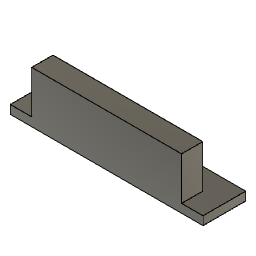
Insert (Autodesk Fusion 360 design; units mm, degrees)
Autodesk Fusion 360 part; units mm, degrees
sketch "Sketch1" plane through (0, 0, 0) normal (0, 0, 1) x (1, 0, 0)
  line L0 (0, 0) -> (44.95, 0)
  line L1 (44.95, 0) -> (44.95, 14.95)
  line L2 (44.95, 14.95) -> (0, 14.95)
  line L3 (0, 14.95) -> (0, 0)
  line L4 (5, 5) -> (39.95, 5)
  line L5 (39.95, 5) -> (39.95, 9.95)
  line L6 (39.95, 9.95) -> (5, 9.95)
  line L7 (5, 9.95) -> (5, 5)
  dimension "d1" = 44.95
  dimension "d2" = 14.95
  dimension "d3" = 34.95
  dimension "d4" = 4.95
  dimension "d5" = 5
  dimension "d6" = 5
  constraint horizontal L0
  constraint vertical L1
  constraint horizontal L2
  constraint vertical L3
  constraint coincident L0.start L3.end
  constraint horizontal L4
  constraint vertical L5
  constraint horizontal L6
  constraint vertical L7
  measures "d1" distance of L0.start L0.end
  measures "d2" distance of L0.start L2.end
  measures "d3" distance of L4.start L4.end
  measures "d4" distance of L4.start L6.end
  measures "d5" distance of L2 L6
  measures "d6" distance of L3 L7
extrude "Extrude1" add sketch "Sketch1" along normal blind 12 contours L4 L5 L6 L7
extrude "Extrude2" add sketch "Sketch1" along normal blind 2
sketch "Sketch2" plane through (0, 0, 2) normal (0, 0, 1) x (-1, 0, 0)
  line L0 (-5, -5) -> (-5, -9.95)
  line L1 (-5, -9.95) -> (-39.95, -9.95)
  line L2 (-39.95, -9.95) -> (-39.95, -5)
  line L3 (-39.95, -5) -> (-5, -5)
  line L4 (0, -14.95) -> (0, 0)
  line L5 (0, 0) -> (-44.95, 0)
  line L6 (-44.95, 0) -> (-44.95, -14.95)
  line L7 (-44.95, -14.95) -> (0, -14.95)
  line L8 (-44.95, 0) -> (0, 0)
  line L9 (0, 0) -> (0, -5)
  line L10 (0, -5) -> (-44.95, -5)
  line L11 (-44.95, -5) -> (-44.95, 0)
  constraint horizontal L8
  constraint vertical L9
  constraint horizontal L10
  constraint vertical L11
  constraint coincident L4 L9.end
  constraint coincident L5.end L6.start
extrude "Extrude3" cut sketch "Sketch2" against normal blind 4 contours L3 L4 L5 L6 L8 L9 L10 L11
